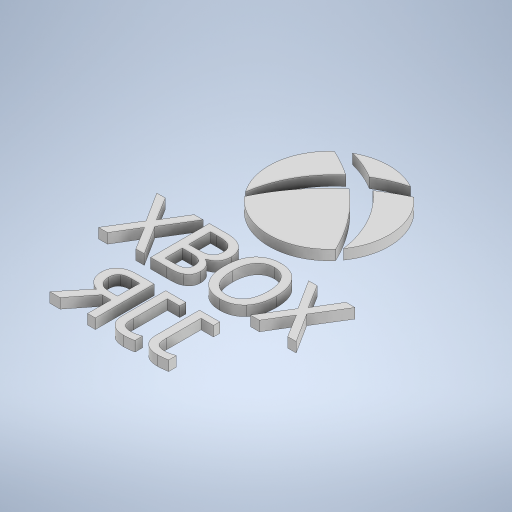
# Autodesk Inventor part: Logotipo
Saved by Autodesk Inventor 2024 (Build 280153000, 153)
## iProperties
Created: 2024-03-05
Part Number: Logotipo
Material: Genérico
Document SubType Name: Modeling
Designer: Juan David
Density: 1 g/cm^3
Appearance: Valor por defecto
Author: Juan David
Autodesk Inventor part; units mm, degrees
ref_plane "YZ Plane" through (0, 0, 0) normal (1, 0, 0) x (0, 1, 0)
ref_plane "XZ Plane" through (0, 0, 0) normal (0, 1, 0) x (-1, 0, 0)
ref_plane "XY Plane" through (0, 0, 0) normal (0, 0, 1) x (1, 0, 0)
sketch "Boceto1" plane through (0, 0, 0) normal (0, 1, 0) x (-1, 0, 0)
  circle A0 centre (0, 0) radius 60
  dimension "d0" = 120
  constraints: 1 centre point, 1 coincident
  measures "d0" diameter of A0
extrude "Extrusión1" add sketch "Boceto1" along normal blind 10
sketch "Boceto3" plane through (0, 10, 0) normal (0, 1, 0) x (1, 0, 0)
  circle A0 centre (0, 0) radius 60 projected
  arc A1 (49, -34.6266) -> (-29, 52.5262) centre (-54.9826, -49.2083) ccw
  line L0 (-29, 52.5262) -> (29, 52.5262)
  line L1 (49, -34.6266) -> (-49, -34.6266)
  arc A2 (29, 52.5262) -> (-49, -34.6266) centre (54.9826, -49.2083) ccw
  arc A3 (45.5961, -39) -> (-39.6863, 45) centre (-112.4424, -114.1589) ccw
  line L2 (-39.6863, 45) -> (39.6863, 45)
  line L3 (45.5961, -39) -> (-45.5961, -39)
  arc A4 (39.6863, 45) -> (-45.5961, -39) centre (112.4424, -114.1589) ccw
  point P0 (-13.6289, 30.2742)
  point P1 (0, 19.937)
  point P2 (13.6289, 30.2742)
  point P3 (0, 40.2451)
  dimension "d15" = 105
  dimension "d16" = 105
  dimension "d17" = 175
  dimension "d18" = 175
  constraints: 8 end point, 8 point on circle, 4 centre point, 3 horizontal, 1 parallel, 9 other
  measures "d15" radius of A1
  measures "d16" radius of A2
  measures "d17" radius of A3
  measures "d18" radius of A4
extrude "Extrusión2" cut sketch "Boceto3" against normal blind 10 contours L2 A2 A0 | A4 A1 A2 L2 | L1 A3 A4 A1 | A0 A3 L1 | A4 A3 A2 A1 | A1 L2 A0 | A2 A3 L2 A1 | A4 L1 A2 A3 | A0 L1 A4
sketch "Boceto4" plane through (0, 0, 0) normal (0, -1, 0) x (1, 0, 0)
  line L0 (0, 0) -> (0, 80)
  line L1 (0, 80) -> (0, 140)
  line L2 (-120, 140) -> (120, 140)
  line L3 (120, 140) -> (120, 80)
  line L4 (120, 80) -> (-120, 80)
  line L5 (-120, 80) -> (-120, 140)
  line L6 (-120, 140) -> (120, 80) construction
  line L7 (120, 140) -> (-120, 80) construction
  line L8 (0, 140) -> (0, 190)
  line L9 (-120, 220) -> (120, 220)
  line L10 (120, 220) -> (120, 160)
  line L11 (120, 160) -> (-120, 160)
  line L12 (-120, 160) -> (-120, 220)
  line L13 (-120, 220) -> (120, 160) construction
  line L14 (120, 220) -> (-120, 160) construction
  line L15 (-92.6891, 140) -> (92.6891, 140) construction
  line L16 (92.6891, 140) -> (92.6891, 78.6947) construction
  line L17 (92.6891, 78.6947) -> (-92.6891, 78.6947) construction
  line L18 (-92.6891, 78.6947) -> (-92.6891, 140) construction
  line L19 (58.4638, 160) -> (-58.4638, 160) construction
  line L20 (-58.4638, 160) -> (-58.4638, 171.4378) construction
  line L21 (-58.4638, 171.4378) -> (58.4638, 171.4378) construction
  line L22 (58.4638, 171.4378) -> (58.4638, 160) construction
  line L23 (-46.0665, 79.9341) -> (-55.0287, 79.9341)
  line L24 (-55.0287, 79.9341) -> (-69.3301, 103.3884)
  line L25 (-69.3301, 103.3884) -> (-83.9175, 79.9341)
  line L26 (-83.9175, 79.9341) -> (-92.3554, 79.9341)
  line L27 (-92.3554, 79.9341) -> (-73.6205, 109.395)
  line L28 (-73.6205, 109.395) -> (-91.7833, 138.7605)
  line L29 (-91.7833, 138.7605) -> (-82.8211, 138.7605)
  line L30 (-82.8211, 138.7605) -> (-68.8057, 115.7353)
  line L31 (-68.8057, 115.7353) -> (-54.5043, 138.7605)
  line L32 (-54.5043, 138.7605) -> (-46.0665, 138.7605)
  line L33 (-46.0665, 138.7605) -> (-64.4677, 109.7764)
  line L34 (-64.4677, 109.7764) -> (-46.0665, 79.9341)
  spline S0 degree 2 poles (0.127, 98.0016) (0.127, 93.6158) (-3.21, 86.8942) (-5.975, 84.7013) knots 0 0 0 1 2 2 2
  spline S1 degree 2 poles (-5.975, 84.7013) (-9.3119, 82.127) (-16.8917, 79.9341) (-22.8983, 79.9341) knots 0 0 0 1 2 2 2
  line L35 (-22.8983, 79.9341) -> (-39.7739, 79.9341)
  line L36 (-39.7739, 79.9341) -> (-39.7739, 138.7605)
  line L37 (-39.7739, 138.7605) -> (-24.1854, 138.7605)
  spline S2 degree 2 poles (-24.1854, 138.7605) (-17.8928, 138.7605) (-11.6002, 137.9501) (-8.7399, 136.377) knots 0 0 0 1 2 2 2
  spline S3 degree 2 poles (-8.7399, 136.377) (-5.5459, 134.7085) (-2.638, 129.2263) (-2.638, 125.5079) knots 0 0 0 1 2 2 2
  spline S4 degree 2 poles (-2.638, 125.5079) (-2.638, 121.3605) (-7.0237, 114.7819) (-10.8851, 112.9227) knots 0 0 0 1 2 2 2
  line L38 (-10.8851, 112.9227) -> (-10.8851, 112.6367)
  spline S5 degree 2 poles (-10.8851, 112.6367) (-5.6413, 111.2065) (0.127, 103.6268) (0.127, 98.0016) knots 0 0 0 1 2 2 2
  spline S6 degree 2 poles (-8.0248, 97.6679) (-8.0248, 101.0049) (-9.9317, 105.2953) (-12.7919, 106.8208) knots 0 0 0 1 2 2 2
  spline S7 degree 2 poles (-12.7919, 106.8208) (-14.6511, 107.7742) (-19.0369, 108.3463) (-23.089, 108.3463) knots 0 0 0 1 2 2 2
  line L39 (-23.089, 108.3463) -> (-31.9558, 108.3463)
  line L40 (-31.9558, 108.3463) -> (-31.9558, 86.6081)
  line L41 (-31.9558, 86.6081) -> (-25.6155, 86.6081)
  spline S8 degree 2 poles (-25.6155, 86.6081) (-20.467, 86.6081) (-14.5558, 87.5616) (-12.2676, 89.087) knots 0 0 0 1 2 2 2
  spline S9 degree 2 poles (-12.2676, 89.087) (-10.0747, 90.6602) (-8.0248, 94.5692) (-8.0248, 97.6679) knots 0 0 0 1 2 2 2
  spline S10 degree 2 poles (-10.7898, 124.4115) (-10.7898, 126.509) (-12.2199, 129.6553) (-13.793, 130.5611) knots 0 0 0 1 2 2 2
  spline S11 degree 2 poles (-13.793, 130.5611) (-15.6999, 131.6099) (-20.324, 132.0866) (-24.4714, 132.0866) knots 0 0 0 1 2 2 2
  line L42 (-24.4714, 132.0866) -> (-31.9558, 132.0866)
  line L43 (-31.9558, 132.0866) -> (-31.9558, 114.8772)
  line L44 (-31.9558, 114.8772) -> (-23.089, 114.8772)
  spline S12 degree 2 poles (-23.089, 114.8772) (-19.4183, 114.8772) (-15.9383, 115.64) (-14.0791, 116.8317) knots 0 0 0 1 2 2 2
  spline S13 degree 2 poles (-14.0791, 116.8317) (-12.2676, 117.9759) (-10.7898, 121.6465) (-10.7898, 124.4115) knots 0 0 0 1 2 2 2
  spline S14 degree 2 poles (49.5145, 132.0389) (52.8514, 128.1298) (56.5698, 116.6887) (56.5698, 109.3473) knots 0 0 0 1 2 2 2
  spline S15 degree 2 poles (56.5698, 109.3473) (56.5698, 102.1967) (52.9468, 90.6125) (49.5145, 86.7035) knots 0 0 0 1 2 2 2
  spline S16 degree 2 poles (49.5145, 86.7035) (45.8914, 82.6037) (36.3095, 78.6947) (30.5413, 78.6947) knots 0 0 0 1 2 2 2
  spline S17 degree 2 poles (30.5413, 78.6947) (24.5824, 78.6947) (15.0481, 82.7468) (11.5681, 86.7035) knots 0 0 0 1 2 2 2
  spline S18 degree 2 poles (11.5681, 86.7035) (8.1834, 90.6125) (4.5604, 102.1013) (4.5604, 109.3473) knots 0 0 0 1 2 2 2
  spline S19 degree 2 poles (4.5604, 109.3473) (4.5604, 116.7364) (8.2311, 127.9868) (11.6158, 132.0389) knots 0 0 0 1 2 2 2
  spline S20 degree 2 poles (11.6158, 132.0389) (15.0481, 135.9479) (24.63, 140) (30.5413, 140) knots 0 0 0 1 2 2 2
  spline S21 degree 2 poles (30.5413, 140) (36.5479, 140) (46.1775, 135.8049) (49.5145, 132.0389) knots 0 0 0 1 2 2 2
  spline S22 degree 2 poles (48.418, 109.3473) (48.418, 115.1632) (45.8914, 124.1731) (43.6032, 127.1287) knots 0 0 0 1 2 2 2
  spline S23 degree 2 poles (43.6032, 127.1287) (41.2673, 130.1797) (34.6887, 133.2307) (30.5889, 133.2307) knots 0 0 0 1 2 2 2
  spline S24 degree 2 poles (30.5889, 133.2307) (26.3462, 133.2307) (19.9582, 130.2751) (17.527, 127.1287) knots 0 0 0 1 2 2 2
  spline S25 degree 2 poles (17.527, 127.1287) (15.1911, 124.1255) (12.7122, 115.0679) (12.7122, 109.3473) knots 0 0 0 1 2 2 2
  spline S26 degree 2 poles (12.7122, 109.3473) (12.7122, 97.7632) (22.4371, 85.464) (30.5889, 85.464) knots 0 0 0 1 2 2 2
  spline S27 degree 2 poles (30.5889, 85.464) (38.7407, 85.464) (48.418, 97.7632) (48.418, 109.3473) knots 0 0 0 1 2 2 2
  line L45 (105.8143, 79.9341) -> (96.8521, 79.9341)
  line L46 (96.8521, 79.9341) -> (82.5507, 103.3884)
  line L47 (82.5507, 103.3884) -> (67.9633, 79.9341)
  line L48 (67.9633, 79.9341) -> (59.5254, 79.9341)
  line L49 (59.5254, 79.9341) -> (78.2603, 109.395)
  line L50 (78.2603, 109.395) -> (60.0975, 138.7605)
  line L51 (60.0975, 138.7605) -> (69.0597, 138.7605)
  line L52 (69.0597, 138.7605) -> (83.0751, 115.7353)
  line L53 (83.0751, 115.7353) -> (97.3765, 138.7605)
  line L54 (97.3765, 138.7605) -> (105.8143, 138.7605)
  line L55 (105.8143, 138.7605) -> (87.4131, 109.7764)
  line L56 (87.4131, 109.7764) -> (105.8143, 79.9341)
  spline S28 degree 2 poles (30.3378, 203.5239) (30.3378, 211.2467) (39.7767, 219.6368) (47.7378, 219.6368) knots 0 0 0 1 2 2 2
  spline S29 degree 2 poles (47.7378, 219.6368) (49.6446, 219.6368) (55.9849, 218.9694) (58.1301, 218.4927) knots 0 0 0 1 2 2 2
  line L57 (58.1301, 218.4927) -> (58.1301, 210.9606)
  line L58 (58.1301, 210.9606) -> (57.7011, 210.9606)
  spline S30 degree 2 poles (57.7011, 210.9606) (56.0803, 211.5327) (51.2655, 212.8675) (48.7866, 212.8675) knots 0 0 0 1 2 2 2
  spline S31 degree 2 poles (48.7866, 212.8675) (45.1635, 212.8675) (40.8254, 211.199) (39.8244, 209.6735) knots 0 0 0 1 2 2 2
  spline S32 degree 2 poles (39.8244, 209.6735) (38.7279, 208.1004) (38.1559, 203.5239) (38.1559, 200.5206) knots 0 0 0 1 2 2 2
  line L59 (38.1559, 200.5206) -> (38.1559, 166.2449)
  line L60 (38.1559, 166.2449) -> (50.5981, 166.2449)
  line L61 (50.5981, 166.2449) -> (50.5981, 160)
  line L62 (50.5981, 160) -> (30.3378, 160)
  line L63 (30.3378, 160) -> (30.3378, 203.5239)
  spline S33 degree 2 poles (-3.3659, 203.5239) (-3.3659, 211.2467) (6.0731, 219.6368) (14.0342, 219.6368) knots 0 0 0 1 2 2 2
  spline S34 degree 2 poles (14.0342, 219.6368) (15.941, 219.6368) (22.2813, 218.9694) (24.4265, 218.4927) knots 0 0 0 1 2 2 2
  line L64 (24.4265, 218.4927) -> (24.4265, 210.9606)
  line L65 (24.4265, 210.9606) -> (23.9975, 210.9606)
  spline S35 degree 2 poles (23.9975, 210.9606) (22.3767, 211.5327) (17.5618, 212.8675) (15.0829, 212.8675) knots 0 0 0 1 2 2 2
  spline S36 degree 2 poles (15.0829, 212.8675) (11.4599, 212.8675) (7.1218, 211.199) (6.1207, 209.6735) knots 0 0 0 1 2 2 2
  spline S37 degree 2 poles (6.1207, 209.6735) (5.0243, 208.1004) (4.4522, 203.5239) (4.4522, 200.5206) knots 0 0 0 1 2 2 2
  line L66 (4.4522, 200.5206) -> (4.4522, 166.2449)
  line L67 (4.4522, 166.2449) -> (16.8945, 166.2449)
  line L68 (16.8945, 166.2449) -> (16.8945, 160)
  line L69 (16.8945, 160) -> (-3.3659, 160)
  line L70 (-3.3659, 160) -> (-3.3659, 203.5239)
  line L71 (-60.4284, 218.8264) -> (-50.2744, 218.8264)
  line L72 (-50.2744, 218.8264) -> (-31.6826, 195.4198)
  line L73 (-31.6826, 195.4198) -> (-22.7204, 195.4198)
  line L74 (-22.7204, 195.4198) -> (-22.7204, 218.8264)
  line L75 (-22.7204, 218.8264) -> (-14.9023, 218.8264)
  line L76 (-14.9023, 218.8264) -> (-14.9023, 160)
  line L77 (-14.9023, 160) -> (-30.0618, 160)
  spline S38 degree 2 poles (-30.0618, 160) (-35.115, 160) (-41.9319, 161.0964) (-45.0306, 163.0986) knots 0 0 0 1 2 2 2
  spline S39 degree 2 poles (-45.0306, 163.0986) (-48.1292, 165.1008) (-51.7046, 171.3458) (-51.7046, 175.9699) knots 0 0 0 1 2 2 2
  spline S40 degree 2 poles (-51.7046, 175.9699) (-51.7046, 182.4055) (-45.1259, 191.1294) (-39.5007, 193.2269) knots 0 0 0 1 2 2 2
  line L78 (-39.5007, 193.2269) -> (-60.4284, 218.8264)
  spline S41 degree 2 poles (-43.5528, 176.5896) (-43.5528, 174.0154) (-41.7413, 170.0586) (-39.8344, 168.7715) knots 0 0 0 1 2 2 2
  spline S42 degree 2 poles (-39.8344, 168.7715) (-38.1659, 167.6751) (-33.7325, 166.7693) (-30.4908, 166.7693) knots 0 0 0 1 2 2 2
  line L79 (-30.4908, 166.7693) -> (-22.7204, 166.7693)
  line L80 (-22.7204, 166.7693) -> (-22.7204, 188.8888)
  line L81 (-22.7204, 188.8888) -> (-29.5851, 188.8888)
  spline S43 degree 2 poles (-29.5851, 188.8888) (-32.9697, 188.8888) (-38.3566, 187.697) (-40.2158, 185.8379) knots 0 0 0 1 2 2 2
  spline S44 degree 2 poles (-40.2158, 185.8379) (-41.9319, 184.217) (-43.5528, 179.6406) (-43.5528, 176.5896) knots 0 0 0 1 2 2 2
  point P0 (0, 110)
  point P1 (0, 140)
  point P2 (0, 160)
  dimension "d21" = 80
  dimension "d22" = 60
  dimension "d23" = 240
  dimension "d24" = 60
  dimension "d25" = 50
  dimension "d26" = 240
  dimension "d27" = 60
  constraints: 30 end point, 9 midpoint, 4 parallel, 2 horizontal, 2 perpendicular, 2 vertical, 1 point on line, 4 other
  measures "d21" distance of L0.start L0.end
  measures "d22" distance of L0.end L1.end
  measures "d23" distance of L3.end L4.end
  measures "d24" distance of L2.end L3.end
  measures "d25" distance of L1.end L8.end
  measures "d26" distance of L10.end L11.end
  measures "d27" distance of L9.end L10.end
extrude "Extrusión3" add sketch "Boceto4" against normal blind 10 contours L11 L70 S33 S34 L64 L65 S35 S36 S37 L66 L67 L68 | S0 S1 L4 L36 L37 S2 S3 S4 L38 S5 L1 | L1 S5 S0 | S17 S18 S19 S20 S21 S14 S15 S16 L4 | L4 S16 S17 | S1 L35 L36 L4 | L49 L50 L51 L52 L53 L54 L55 L56 L4 L46 L47 | L4 L47 L48 L49 | L34 L23 L24 L4 | L4 L24 L25 L27 L28 L29 L30 L31 L32 L33 L34 | L4 L56 L45 L46 | L25 L26 L27 L4 | L63 S28 S29 L57 L58 S30 S31 S32 L59 L60 L61 L11 | L11 S38 S39 S40 L78 L71 L72 L73 L74 L75 L76
